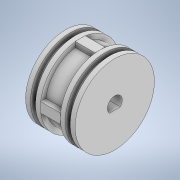
# Autodesk Inventor part: lepszy kolo
Saved by Autodesk Inventor 2020 (Build 240168000, 168)
## iProperties
Created: 2023-03-02
Part Number: lepszy kolo
Material: Ogólny
Document SubType Name: Modeling
Designer: User
Density: 1 g/cm^3
Appearance: Domyślna
Author: User
Autodesk Inventor part; units mm, degrees
ref_plane "YZ Plane" through (0, 0, 0) normal (1, 0, 0) x (0, 1, 0)
ref_plane "XZ Plane" through (0, 0, 0) normal (0, 1, 0) x (-1, 0, 0)
ref_plane "XY Plane" through (0, 0, 0) normal (0, 0, 1) x (1, 0, 0)
sketch "Szkic1" plane through (0, 0, 0) normal (1, 0, 0) x (0, 1, 0)
  circle A0 centre (0, 0) radius 7
  circle A1 centre (0, 0) radius 1.5
  line L0 (0, 1.5) -> (0, -1.0846)
  line L1 (-1, 1.9718) -> (-1, -1.0846)
  line L2 (8, 0) -> (-8, 0)
  line L3 (-8, 0) -> (-8, -1)
  line L4 (-8, -1) -> (8, -1)
  line L5 (8, -1) -> (8, 0)
  line L6 (8, 0) -> (-8, 0)
  line L7 (-8, 0) -> (-8, 1)
  line L8 (-8, 1) -> (8, 1)
  line L9 (8, 1) -> (8, 0)
  line L10 (0, 8) -> (1, 8)
  line L11 (1, 8) -> (1, -8)
  line L12 (1, -8) -> (0, -8)
  line L13 (0, 8) -> (-1, 8)
  line L14 (-1, 8) -> (-1, -8)
  line L15 (-1, -8) -> (0, -8)
  line L16 (0, -8) -> (0, 8)
  point P0 (-1, -1.118)
  point P1 (-1, 1.118)
  point P2 (-6.9282, -1)
  point P3 (-6.9282, 1)
  point P4 (1, -6.9282)
  point P5 (-1, -6.9282)
  point P6 (6.9282, 1)
  point P7 (6.9282, -1)
  point P8 (-1, 6.9282)
  point P9 (1, 6.9282)
  dimension "d1" = 3
  dimension "d0" = 14
  dimension "d2" = 1
  dimension "d14" = 16
  dimension "d16" = 16
  dimension "d18" = 2
  dimension "d19" = 2
  constraints: 34 end point, 7 parallel, 4 horizontal, 4 perpendicular, 3 coincident, 2 midpoint, 2 vertical, 1 centre point, 9 other
  measures "d0" diameter of A0
  measures "d2" distance between parallel lines of L1 L0
  measures "d14" distance of L3.end L4.end
  measures "d16" distance of L10.end L11.end
  measures "d18" distance between parallel lines of L14 L11
  measures "d19" distance between parallel lines of L4 L8
sketch "Szkic2" plane through (0, 0, 0) normal (0, 0, 1) x (1, 0, 0)
  line L0 (0, 0) -> (5, 0)
  line L1 (5, 0) -> (5, 7)
  line L2 (5, 7) -> (0, 7)
  line L3 (0, 7) -> (0, 0)
  line L4 (0, 0) -> (-5, 0)
  line L5 (-5, 0) -> (-5, 7)
  line L6 (-5, 7) -> (0, 7)
  line L7 (0, 7) -> (0, 0)
  line L8 (0, 0) -> (5, 0)
  line L9 (5, 0) -> (5, -7)
  line L10 (5, -7) -> (0, -7)
  line L11 (0, -7) -> (0, 0)
  line L12 (0, 0) -> (-5, 0)
  line L13 (-5, 0) -> (-5, -7)
  line L14 (-5, -7) -> (0, -7)
  line L15 (0, -7) -> (0, 0)
  line L16 (5, 7) -> (4, 7)
  line L17 (4, 7) -> (4, 8)
  line L18 (4, 8) -> (5, 8)
  line L19 (5, 8) -> (5, 7)
  line L20 (3, 7) -> (2, 7)
  line L21 (2, 7) -> (2, 8)
  line L22 (2, 8) -> (3, 8)
  line L23 (3, 8) -> (3, 7)
  line L24 (-5, 7) -> (-4, 7)
  line L25 (-4, 7) -> (-4, 8)
  line L26 (-4, 8) -> (-5, 8)
  line L27 (-5, 8) -> (-5, 7)
  line L28 (-3, 7) -> (-2, 7)
  line L29 (-2, 7) -> (-2, 8)
  line L30 (-2, 8) -> (-3, 8)
  line L31 (-3, 8) -> (-3, 7)
  dimension "d3" = 5
  dimension "d4" = 7
  dimension "d5" = 10
  dimension "d6" = 14
  dimension "d7" = 1
  dimension "d8" = 1
  dimension "d9" = 1
  dimension "d10" = 1
  dimension "d11" = 1
  dimension "d12" = 1
  dimension "d13" = 1
  constraints: 64 end point, 16 parallel, 8 horizontal, 8 perpendicular, 2 point on line
  measures "d3" distance of L1.end L2.end
  measures "d4" distance of L0.end L1.end
  measures "d5" distance between parallel lines of L1 L5
  measures "d6" distance between parallel lines of L10 L2
  measures "d7" distance of L17.end L18.end
  measures "d8" distance of L18.end L1.end
  measures "d9" distance of L21.end L22.end
  measures "d10" distance of L25.end L26.end
  measures "d11" distance between parallel lines of L17 L23
  measures "d12" distance of L29.end L30.end
  measures "d13" distance between parallel lines of L31 L25
extrude "Wyciągnięcie proste1" add sketch "Szkic1" along normal mid plane 10 contours L2 A1 L8 A0 | A0 L4 A1 L2 | L8 A1 L11 A0 | A0 L11 A1 L4 | L11 A1 L16 A0 | A0 L16 A1 L11 | L16 A1 L1 L14 A0 | A0 L14 A1 L16 | L14 L1 A1 L8 A0 | A0 L4 A1 L14 | L2 A1 L8 L1 | L1 L4 A1 L2 | L8 A1 L2 A0 | L1 L8 A1 | A0 L2 A1 L4 | A1 L4 L1 L14
extrude "Wyciągnięcie proste2" add sketch "Szkic1" along normal mid plane 4 contours L2 L5 L4 A0 | A0 L8 L9 L2 | A0 L16 L10 L11 | L11 L12 L16 A0 | A0 L14 L13 L16 | L16 L15 L14 A0 | A0 L2 L7 L8 | L4 L3 L2 A0
revolve "Obrót1" add sketch "Szkic2" angle 360 about axis through (0, 0, 0) along (1, 0, 0) contours L2 L17 L18 L19 | L21 L22 L23 L2 | L6 L31 L30 L29 | L27 L26 L25 L6
